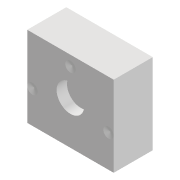
# Autodesk Inventor part: 10_SOOCT_VCM_Mount_v0
Saved by Autodesk Inventor 2022 (Build 260153000, 153)
## iProperties
Created: 2023-01-02
Part Number: 10_SOOCT_VCM_Mount_v0
Material: Generisch
Document SubType Name: Modeling
Designer: diederichbenedict
Density: 1 g/cm^3
Appearance: Vorgabe
Author: diederichbenedict
Autodesk Inventor part; units mm, degrees
ref_plane "YZ Plane" through (0, 0, 0) normal (1, 0, 0) x (0, 1, 0)
ref_plane "XZ Plane" through (0, 0, 0) normal (0, 1, 0) x (-1, 0, 0)
ref_plane "XY Plane" through (0, 0, 0) normal (0, 0, 1) x (1, 0, 0)
sketch "Skizze1" plane through (0, 0, 0) normal (0, 0, 1) x (1, 0, 0)
  arc A0 (-9, -8) -> (-8, -9) centre (-8, -8) ccw projected
  line L0 (8, -9) -> (-8, -9) projected
  arc A1 (8, -9) -> (9, -8) centre (8, -8) ccw projected
  line L1 (9, 8) -> (9, -8) projected
  arc A2 (9, 8) -> (8, 9) centre (8, 8) ccw projected
  line L2 (-8, 9) -> (8, 9) projected
  arc A3 (-8, 9) -> (-9, 8) centre (-8, 8) ccw projected
  line L3 (-9, -8) -> (-9, 8) projected
  circle A4 centre (0, 0) radius 5.8 projected
  arc A5 (-8, 9.1) -> (-9.1, 8) centre (-8, 8) ccw
  line L4 (-8, 9.1) -> (8, 9.1)
  arc A6 (9.1, 8) -> (8, 9.1) centre (8, 8) ccw
  line L5 (9.1, 8) -> (9.1, -8)
  arc A7 (8, -9.1) -> (9.1, -8) centre (8, -8) ccw
  line L6 (8, -9.1) -> (-8, -9.1)
  arc A8 (-9.1, -8) -> (-8, -9.1) centre (-8, -8) ccw
  line L7 (-9.1, -8) -> (-9.1, 8)
  line L8 (14, 14) -> (-14, 14)
  line L9 (-14, 14) -> (-14, -14)
  line L10 (-14, -14) -> (14, -14)
  line L11 (14, -14) -> (14, 14)
  line L12 (14, 14) -> (-14, -14) construction
  line L13 (-14, 14) -> (14, -14) construction
  point P0 (0, 0)
  dimension "d0" = 0.1
  dimension "d1" = 28
  dimension "d2" = 28
  constraints: 20 end point, 8 point on circle, 4 centre point, 2 midpoint, 2 parallel, 1 horizontal, 1 perpendicular, 7 other
  measures "d0" distance between parallel lines of L3 L7
  measures "d1" distance of L10.end L9.end
  measures "d2" distance of L9.end L8.end
ref_plane "Arbeitsebene1" through (-9, -9, -7.8) normal (0, 0, -1) x (0, 1, 0)
extrude "Extrusion1" add sketch "Skizze1" against normal up to surface (7.8 mm away) contours L11 L10 L9 L8
sketch "Skizze2" plane through (0, 0, 0) normal (0, 0, 1) x (1, 0, 0)
  line L0 (-14, 14) -> (-14, -14) projected
  line L1 (-14, -14) -> (14, -14) projected
  line L2 (14, -14) -> (14, 14) projected
  line L3 (14, 14) -> (-14, 14) projected
  line L4 (9.1, 8) -> (9.1, -8) projected
  arc A0 (8, -9.1) -> (9.1, -8) centre (8, -8) ccw projected
  line L5 (8, -9.1) -> (-8, -9.1) projected
  arc A1 (-9.1, -8) -> (-8, -9.1) centre (-8, -8) ccw projected
  line L6 (-9.1, -8) -> (-9.1, 8) projected
  arc A2 (-8, 9.1) -> (-9.1, 8) centre (-8, 8) ccw projected
  line L7 (-8, 9.1) -> (8, 9.1) projected
  arc A3 (9.1, 8) -> (8, 9.1) centre (8, 8) ccw projected
  line L8 (-7.6, 7.6) -> (-7.6, -7.6)
  line L9 (-7.6, -7.6) -> (7.6, -7.6)
  line L10 (7.6, -7.6) -> (7.6, 7.6)
  line L11 (7.6, 7.6) -> (-7.6, 7.6)
  point P0 (0, 0)
  dimension "d5" = 1.5
  constraints: 8 end point, 3 other
  measures "d5" distance between parallel lines of L6 L8
extrude "Extrusion2" add sketch "Skizze2" along normal blind 0.5 contours L3 L2 L1 L0 | L4 A0 L5 A1 L6 A2 L7 A3 | L11 L10 L9 L8
sketch "Skizze3" plane through (0, 0, 0.5) normal (0, 0, 1) x (1, 0, 0)
  line L0 (-14, -14) -> (14, -14) projected
  line L1 (14, -14) -> (14, 14) projected
  line L2 (14, 14) -> (-14, 14) projected
  line L3 (-14, 14) -> (-14, -14) projected
  circle A0 centre (0, 3.1887) radius 4
  dimension "d8" = 8
  constraints: 1 centre point
  measures "d8" diameter of A0
extrude "Extrusion3" add sketch "Skizze3" along normal blind 3
sketch "Skizze4" plane through (0, 0, 3.5) normal (0, 0, 1) x (1, 0, 0)
  line L0 (14, -14) -> (14, 14) projected
  line L1 (14, 14) -> (-14, 14) projected
  line L2 (-14, 14) -> (-14, -14) projected
  line L3 (-14, -14) -> (14, -14) projected
  circle A0 centre (0, 3.1887) radius 4 projected
  line L4 (5, -10.8) -> (-5, -10.8) projected
  line L5 (-14, 14) -> (-14, -14) projected
  line L6 (14, -14) -> (-14, -14)
  line L7 (-14, -14) -> (-14, -9.3)
  line L8 (-14, -9.3) -> (14, -9.3)
  line L9 (14, -9.3) -> (14, -14)
  line L10 (-14, 14) -> (-12.5, 14)
  line L11 (-12.5, 14) -> (-12.5, -9.3)
  line L12 (-12.5, -9.3) -> (-14, -9.3)
  line L13 (-14, -9.3) -> (-14, 14)
  line L14 (14, -14) -> (14, 14) projected
  line L15 (14, 14) -> (12.5, 14)
  line L16 (12.5, 14) -> (12.5, -9.3)
  line L17 (12.5, -9.3) -> (14, -9.3)
  line L18 (14, -9.3) -> (14, 14)
  point P0 (0, 0)
  point P1 (14, -9.3)
  point P2 (12.5, 14)
  dimension "d11" = 1.5
  dimension "d22" = 1.5
  dimension "d23" = 1.5
  constraints: 24 end point, 6 parallel, 3 horizontal, 3 perpendicular, 3 point on line
  measures "d11" distance from line of L8 L4.start
  measures "d22" distance of L11.end L12.end
  measures "d23" distance of L17.end L16.end
extrude "Extrusion4" cut sketch "Skizze4" against normal through all contours L3 L2 L8 L0 | L8 L16 L1 L0 | L2 L1 L11 L8
sketch "Skizze5" plane through (0, 0, 3.5) normal (0, 0, 1) x (1, 0, 0)
  circle A0 centre (0, 0) radius 5.8 projected
  circle A1 centre (0, 0) radius 11 construction
  point P0 (0, 0)
  point P1 (-11, 0)
  point P2 (11, 0)
  point P3 (0, 11)
  dimension "d14" = 22
  constraints: 3 point on circle, 1 centre point, 1 coincident
  measures "d14" diameter of A1
hole "Bohrung1" at (-11, 0, 3.5) at (11, 0, 3.5) at (0, 11, 3.5) direction (0, 0, -1) diameter 3 depth 0.0001 tip angle 140
